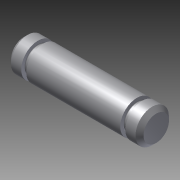
# Autodesk Inventor part: D-25368
Saved by Autodesk Inventor 2012 (Build 160160000, 160)
## iProperties
Created: 2013-01-17
Part Number: D-25368
Material: Default
Catalog Web Link: www.cadenas.de
Description: Piston Rod Clevis for Original Line Cylinders - Pin-
Vendor: BIMBA
Document SubType Name: Modeling
Designer: William
Manufacturer: BIMBA
Density: 1 g/cm^3
Category: PARTsolutions
Company: BIMBA
Title: D-25368
Author: Cadenas PARTsolutions
PSOL_IDENT_0: {\\10.0.0.242\data_v9\23d-libs\bimba\bimba\bimba_imperial\bimba_full_line\original_line_cylinders\ac
PSOL_IDENT_1: cessories\piston_rod_clevis_pin.prj},201 {VTYP=3D},{NB=D-25368},{LINA=D-25368},{NN=Piston Rod Clevis
PSOL_IDENT_2: for Original Line Cylinders - Pin},{DATE=06.12.2012 07:28:06},{GEOMDATE=06.12.2012 07:18:17},{VERSI
PSOL_IDENT_3: ON=},{LINEID=10},{LINESUBID=-1},{WBVAR=}  {NB=D-25368},{LINA=D-25368},{KT=DUMMY},{PN=D-25368},{L=0.4
PSOL_IDENT_4: 9500000},{L1=0.35100000},{L2=0.01900000},{L4=0.06600000},{D=0.12500000},{D1=0.09600000},{CH=0.015000
PSOL_IDENT_5: 00},{R=0.00250000},{COLOR=0.75,0.75,0.75,0.00}
CNS_NB: D-25368
CNS_NBSYN: $PN.
CNS_LINA: D-25368
CNS_PN: D-25368
CNS_L: 0.49500000
CNS_L1: 0.35100000
CNS_L2: 0.01900000
CNS_L4: 0.06600000
CNS_D: 0.12500000
CNS_D1: 0.09600000
CNS_CH: 0.01500000
CNS_R: 0.00250000
CNS_COLOR: 0.75,0.75,0.75,0.00
SUPPLIER: BIMBA
ARTICLENO: D-25368
BOMINFO: D-25368
CREATOR: CADENAS GmbH
Autodesk Inventor part; units mm, degrees
sketch "Sketch_1" plane through (0, 0, 0) normal (0, 0, 1) x (1, 0, 0)
  line L0 (6.2865, 0) -> (-6.2865, 0)
  line L1 (-6.2865, 0) -> (-6.2865, 1.2065)
  line L2 (-6.2865, 1.2065) -> (-5.9055, 1.5875)
  line L3 (-5.9055, 1.5875) -> (-4.9403, 1.5875)
  line L4 (-4.9403, 1.5875) -> (-4.9403, 1.2827)
  arc A0 (-4.9403, 1.2827) -> (-4.8768, 1.2192) centre (-4.8768, 1.2827) ccw
  line L5 (-4.8768, 1.2192) -> (-4.5212, 1.2192)
  arc A1 (-4.5212, 1.2192) -> (-4.4577, 1.2827) centre (-4.5212, 1.2827) ccw
  line L6 (-4.4577, 1.2827) -> (-4.4577, 1.5875)
  line L7 (-4.4577, 1.5875) -> (4.4577, 1.5875)
  line L8 (4.4577, 1.5875) -> (4.4577, 1.2827)
  arc A2 (4.4577, 1.2827) -> (4.5212, 1.2192) centre (4.5212, 1.2827) ccw
  line L9 (4.5212, 1.2192) -> (4.8768, 1.2192)
  arc A3 (4.8768, 1.2192) -> (4.9403, 1.2827) centre (4.8768, 1.2827) ccw
  line L10 (4.9403, 1.2827) -> (4.9403, 1.5875)
  line L11 (4.9403, 1.5875) -> (5.9055, 1.5875)
  line L12 (5.9055, 1.5875) -> (6.2865, 1.2065)
  line L13 (6.2865, 1.2065) -> (6.2865, 0)
  line L14 (6.2865, 0) -> (-6.2865, 0)
  constraints: 30 end point, 8 point on circle, 4 centre point
revolve "Revolution1" add sketch "Sketch_1" angle 360 about axis through (6.2865, 0, 0) along (1, 0, 0)
ref_plane "pin_XY" through (0, 0, 0) normal (1, 0, 0) x (0, 0, -1)
ref_plane "pin_YZ" through (0, 0, 0) normal (0, 0, -1) x (0, 1, 0)
ref_plane "pin_ZX" through (0, 0, 0) normal (0, 1, 0) x (1, 0, 0)
ref_plane "rr1_XY" through (4.699, 0, 0) normal (1, 0, 0) x (0, 0, -1)
ref_plane "rr1_YZ" through (4.699, 0, 0) normal (0, 0, -1) x (0, 1, 0)
ref_plane "rr1_ZX" through (4.699, 0, 0) normal (0, 1, 0) x (1, 0, 0)
ref_plane "rr2_XY" through (-4.699, 0, 0) normal (1, 0, 0) x (0, 0, -1)
ref_plane "rr2_YZ" through (-4.699, 0, 0) normal (0, 0, -1) x (0, 1, 0)
ref_plane "rr2_ZX" through (-4.699, 0, 0) normal (0, 1, 0) x (1, 0, 0)
ref_plane "w21_XY" through (6.2865, 0, 0) normal (0, 1, 0) x (1, 0, 0)
ref_plane "w21_YZ" through (6.2865, 0, 0) normal (1, 0, 0) x (0, 0, -1)
ref_plane "w21_ZX" through (6.2865, 0, 0) normal (0, 0, -1) x (0, 1, 0)
ref_plane "w22_XY" through (-6.2865, 0, 0) normal (0, 1, 0) x (1, 0, 0)
ref_plane "w22_YZ" through (-6.2865, 0, 0) normal (1, 0, 0) x (0, 0, -1)
ref_plane "w22_ZX" through (-6.2865, 0, 0) normal (0, 0, -1) x (0, 1, 0)
ref_plane "p1_XY" through (0, 0, 1.5875) normal (1, 0, 0) x (0, 0, -1)
ref_plane "p1_YZ" through (0, 0, 1.5875) normal (0, 0, -1) x (0, 1, 0)
ref_plane "p1_ZX" through (0, 0, 1.5875) normal (0, 1, 0) x (1, 0, 0)
ref_plane "p2_XY" through (0, 0, -1.5875) normal (1, 0, 0) x (0, 0, -1)
ref_plane "p2_YZ" through (0, 0, -1.5875) normal (0, 0, -1) x (0, 1, 0)
ref_plane "p2_ZX" through (0, 0, -1.5875) normal (0, 1, 0) x (1, 0, 0)
body "Solid1"
